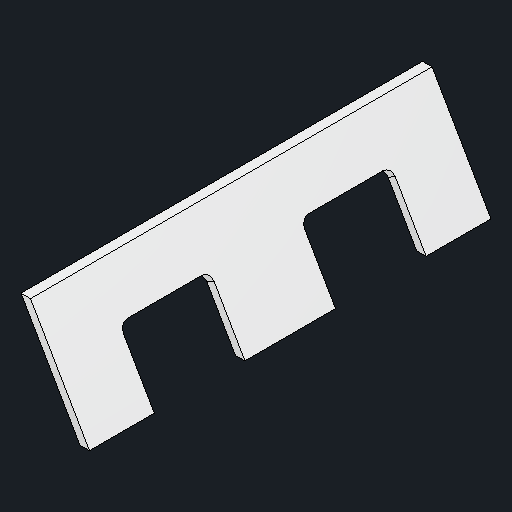
# Autodesk Inventor part: Przod
Saved by Autodesk Inventor 2023 (Build 270158000, 158)
## iProperties
Created: 2024-02-26
Part Number: Przod
Material: Aluminum 6061
Document SubType Name: Modeling
Designer: Michał
Density: 2.7 g/cm^3
Appearance: Aluminum - Flat
Author: Michał
Autodesk Inventor part; units mm, degrees
ref_plane "YZ Plane" through (0, 0, 0) normal (1, 0, 0) x (0, 1, 0)
ref_plane "XZ Plane" through (0, 0, 0) normal (0, 1, 0) x (-1, 0, 0)
sketch "Sketch1" plane through (0, 0, 0) normal (0, 0, 1) x (1, 0, 0)
  line L0 (44.9961, 27) -> (47.3055, 27)
  line L1 (47.3055, 27) -> (61.6238, 2.2)
  line L2 (61.6238, 2.2) -> (59.3144, 2.2)
  line L3 (59.3144, 2.2) -> (44.9961, 27) construction
  line L4 (44.9961, 27) -> (59.3144, 2.2)
  line L5 (16.5, 27) -> (44.9961, 27) construction
  point P0 (0, 0)
  dimension "d10" = 2
  constraints: 12 end point, 2 equal length, 2 horizontal, 1 collinear, 1 point on line, 4 other
  measures "d10" distance between parallel lines of L1 L3
ref_plane "Work Plane1" through (0, 0, -97.5) normal (0, 0, -1) x (0, 1, 0)
extrude "Extrusion1" add sketch "Sketch1" against normal up to surface (97.5 mm away)
sketch "Sketch2" plane through (47.3055, 27, 0) normal (0.8660254, 0.5, 0) x (0, 0, -1)
  line L0 (15.75, -28.6366) -> (37.75, -28.6366)
  line L1 (37.75, -28.6366) -> (37.75, -11.6366)
  line L2 (37.75, -11.6366) -> (15.75, -11.6366)
  line L3 (15.75, -11.6366) -> (15.75, -28.6366)
  line L4 (0, 0) -> (97.5, 0) construction
  line L5 (48.75, 0) -> (48.75, -28.6366) construction
  line L6 (0, -28.6366) -> (97.5, -28.6366) construction
  line L7 (81.75, -28.6366) -> (59.75, -28.6366)
  line L8 (59.75, -28.6366) -> (59.75, -11.6366)
  line L9 (59.75, -11.6366) -> (81.75, -11.6366)
  line L10 (81.75, -11.6366) -> (81.75, -28.6366)
  point P0 (0, 0.2701)
  dimension "d4" = 22
  dimension "d5" = 22
  dimension "d6" = 17
  constraints: 18 end point, 4 symmetric about line, 2 midpoint, 2 parallel, 1 collinear, 1 horizontal, 1 perpendicular
  measures "d4" distance between parallel lines of L1 L3
  measures "d5" diameter of L1 L5
  measures "d6" distance between parallel lines of L0 L2
extrude "Extrusion2" cut sketch "Sketch2" against normal through all
fillet "Fillet1" radius 2 4 edges at (52.2577, 16.4224, -37.75) (52.2577, 16.4224, -15.75) (52.2577, 16.4224, -59.75) (52.2577, 16.4224, -81.75)
body "Solid1"
